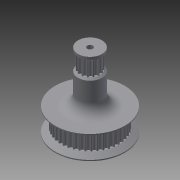
# Autodesk Inventor part: gates 42 pulley and gates 15 pulley
Saved by Autodesk Inventor 2015 (Build 190159000, 159)
## iProperties
Created: 2015-02-13
Part Number: gates 42 pulley and gates 15 pulley
Material: Generic
Document SubType Name: Modeling
Designer: robotics
Density: 1 g/cm^3
Appearance: Default
Author: robotics
Autodesk Inventor part; units mm, degrees
ref_plane "YZ Plane" through (0, 0, 0) normal (1, 0, 0) x (0, 1, 0)
ref_plane "XZ Plane" through (0, 0, 0) normal (0, 1, 0) x (-1, 0, 0)
ref_plane "XY Plane" through (0, 0, 0) normal (0, 0, 1) x (1, 0, 0)
sketch "Sketch1" plane through (0, 0, 0) normal (0, 1, 0) x (-1, 0, 0)
  circle A0 centre (0, 0) radius 32.766
  dimension "d0" = 65.532
  constraints: 1 centre point, 1 coincident
  measures "d0" diameter of A0
extrude "Extrusion1" add sketch "Sketch1" along normal blind 16.51
sketch "Sketch2" plane through (0, 16.51, 0) normal (0, 1, 0) x (1, 0, 0)
  circle A0 centre (0, 0) radius 32.766 construction
  circle A1 centre (0, 0) radius 30.6832 construction
  line L0 (0, 0) -> (-47.2853, 0) construction
  line L1 (0, 0) -> (-30.5974, -2.293) construction
  line L2 (0, 0) -> (-30.5974, 2.293) construction
  line L3 (-32.766, -0.6731) -> (-32.766, 0.6731)
  line L4 (-32.766, -0.6731) -> (-30.6758, -0.6731) construction
  line L5 (-32.766, 0.6731) -> (-32.3432, 0.6731)
  circle A2 centre (-32.3432, -2.4238) radius 1.7507 construction
  circle A3 centre (-32.3432, 2.4238) radius 1.7507 construction
  line L6 (-32.5004, 4.2179) -> (-32.2997, 5.5491)
  line L7 (-32.5004, 4.2179) -> (-32.0823, 4.1549)
  arc A4 (-32.3432, 0.6731) -> (-32.0823, 4.1549) centre (-32.3432, 2.4238) ccw
  arc A5 (-32.5004, 4.2179) -> (-32.766, 0.6731) centre (0, 0) ccw
  point P0 (-32.4, 4.8835)
  dimension "d3" = 65.532
  dimension "d4" = 61.3664
  dimension "d5" = 8.571
  dimension "d6" = 1.3462
  constraints: 16 end point, 9 point on circle, 5 centre point, 4 coincident, 4 tangent, 3 horizontal, 2 line through centre, 2 vertical, 1 equal length, 1 equal radius, 1 midpoint, 1 perpendicular, 1 symmetric about line, 5 other
  measures "d4" diameter of A1
  measures "d5" angle of L2 L1
  measures "d6" distance of L3.start L3.end
extrude "Extrusion2" cut sketch "Sketch2" against normal through all
fillet "Fillet1" radius 0.127 2 edges at (-32.7591, 8.255, -0.6731) (-32.4935, 8.255, -4.2169)
pattern_circular "Circular Pattern1" count 42 over 360 about axis through (0, 0, 0) along (0, 1, 0) of "Extrusion2", "Fillet1"
sketch "Sketch3" plane through (0, 0, 0) normal (0, 0, 1) x (1, 0, 0)
  line L0 (0, 0) -> (32.766, 0)
  line L1 (32.766, 0) -> (39.116, -3.81)
  line L2 (39.116, -3.81) -> (39.116, -4.953)
  line L3 (39.116, -4.953) -> (0, -4.953)
  line L4 (0, -4.953) -> (0, 0)
  line L5 (-1.7458, 16.51) -> (1.7458, 16.51) projected
  line L6 (0, 16.51) -> (32.766, 16.51)
  line L7 (32.766, 16.51) -> (39.116, 20.32)
  line L8 (39.116, 20.32) -> (39.116, 21.463)
  line L9 (0, 57.15) -> (0, 16.51)
  line L10 (0, 57.15) -> (11.3665, 57.15)
  line L11 (11.3665, 57.15) -> (13.4747, 55.372)
  line L12 (13.4747, 55.372) -> (13.4747, 51.0934)
  line L13 (13.4747, 51.0934) -> (13.4747, 21.463)
  line L14 (13.4747, 21.463) -> (39.116, 21.463)
  dimension "d13" = 32.766
  dimension "d14" = 3.81
  dimension "d15" = 6.35
  dimension "d16" = 4.953
  dimension "d17" = 32.766
  dimension "d18" = 3.81
  dimension "d19" = 6.35
  dimension "d22" = 4.953
  dimension "d23" = 62.103
  dimension "d24" = 11.3665
  dimension "d26" = 1.778
  dimension "d27" = 2.1082
  dimension "d54" = 13.4747
  dimension "d55" = 39.116
  constraints: 28 end point, 5 perpendicular, 2 horizontal, 1 collinear, 1 midpoint, 1 point on line, 1 vertical
  measures "d13" distance of L0.start L0.end
  measures "d14" vertical distance of L1.end L0.end
  measures "d15" horizontal distance of L1.end L0.end
  measures "d16" distance of L3.end L0.start
  measures "d17" distance of L6.start L6.end
  measures "d18" vertical distance of L7.end L6.end
  measures "d19" horizontal distance of L6.end L7.end
  measures "d22" vertical distance of L8.end L6.end
  measures "d23" distance of L9.start L3.end
  measures "d24" distance of L9.start L10.end
  measures "d26" vertical distance of L10.end L11.end
  measures "d27" horizontal distance of L10.end L11.end
  measures "d54" distance between parallel lines of L13 L9
  measures "d55" distance of L2.end L3.end
revolve "Revolution1" add sketch "Sketch3" angle 360 about axis through (0, 57.15, 0) along (0, -1, 0)
fillet "Fillet2" radius 12.7 1 edges at (-13.4747, 21.463, 0)
sketch "Sketch5" plane through (0, 57.15, 0) normal (0, 1, 0) x (1, 0, 0)
  circle A0 centre (0, 0) radius 11.3665
  dimension "d33" = 22.733
  constraints: 1 centre point, 1 coincident
  measures "d33" diameter of A0
extrude "Extrusion3" add sketch "Sketch5" along normal blind 16.51
sketch "Sketch6" plane through (0, 73.66, 0) normal (0, 1, 0) x (1, 0, 0)
  circle A0 centre (0, 0) radius 11.3665 construction
  circle A1 centre (0, 0) radius 9.2837 construction
  line L0 (0, 0) -> (0, 14.8033) construction
  line L1 (0, 0) -> (-1.9302, 9.0808) construction
  line L2 (0, 0) -> (1.9302, 9.0808) construction
  line L3 (-0.6731, 11.3665) -> (0.6731, 11.3665)
  circle A2 centre (-2.2602, 10.6332) radius 1.5871 construction
  circle A3 centre (2.2602, 10.6332) radius 1.5871 construction
  line L4 (-0.6731, 11.3665) -> (-0.6731, 9.2593) construction
  line L5 (0.6731, 11.3665) -> (0.6731, 10.6332)
  line L6 (4.0083, 10.6576) -> (5.2381, 10.11)
  line L7 (4.0083, 10.6576) -> (3.71, 9.9877)
  circle A4 centre (0, 0) radius 11.3665 construction
  arc A5 (0.6731, 10.6332) -> (3.71, 9.9877) centre (2.2602, 10.6332) ccw
  arc A6 (4.0083, 10.6576) -> (0.6731, 11.3665) centre (0.9264, 4.3583) ccw
  point P0 (4.6232, 10.3838)
  dimension "d36" = 22.733
  dimension "d37" = 18.5674
  dimension "d38" = 24
  dimension "d39" = 1.3462
  constraints: 16 end point, 9 point on circle, 6 centre point, 5 tangent, 3 coincident, 3 vertical, 2 line through centre, 1 equal length, 1 equal radius, 1 horizontal, 1 midpoint, 1 perpendicular, 1 symmetric about line, 4 other
  measures "d36" diameter of A0
  measures "d37" diameter of A1
  measures "d38" angle of L2 L1
  measures "d39" distance of L3.start L3.end
extrude "Extrusion4" cut sketch "Sketch6" against normal blind 16.51
fillet "Fillet3" radius 0.127 2 edges at (4.0002, 65.405, -10.6394) (0.6731, 65.405, -11.3466)
pattern_circular "Circular Pattern2" count 15 over 360 about axis through (0, 57.15, 0) along (0, 1, 0) of "Extrusion4", "Fillet3"
sketch "Sketch7" plane through (0, 0, 0) normal (0, 0, 1) x (1, 0, 0)
  line L0 (-1.5524, 73.66) -> (1.5524, 73.66) projected
  line L1 (0, 73.66) -> (11.3665, 73.66)
  line L2 (7.8273, 73.66) -> (9.9048, 73.66) projected
  line L3 (11.3665, 73.66) -> (13.4747, 75.438)
  line L4 (13.4747, 75.438) -> (13.4747, 78.613)
  line L5 (13.4747, 78.613) -> (0, 78.613)
  line L6 (0, 78.613) -> (0, 73.66)
  point P0 (0, 0)
  point P1 (8.3524, 73.66)
  dimension "d46" = 11.3665
  dimension "d47" = 1.778
  dimension "d48" = 2.1082
  dimension "d49" = 3.175
  constraints: 10 end point, 3 perpendicular, 1 collinear, 1 midpoint
  measures "d46" distance of L1.start L1.end
  measures "d47" vertical distance of L3.end L1.end
  measures "d48" horizontal distance of L1.end L3.end
  measures "d49" distance of L3.end L4.end
revolve "Revolution2" add sketch "Sketch7" angle 360 about axis through (0, 78.613, 0) along (0, -1, 0)
sketch "Sketch8" plane through (0, 78.613, 0) normal (0, 1, 0) x (1, 0, 0)
  circle A0 centre (0, 0) radius 3.175
  dimension "d51" = 6.35
  constraints: 1 centre point, 1 coincident
  measures "d51" diameter of A0
extrude "Extrusion5" cut sketch "Sketch8" against normal through all
equation "\"d13\" = 0.5 * d0"
equation "\"d17\" = 0.5 * d0"
equation "\"d18\" = d14"
equation "\"d19\" = d15"
equation "\"d22\" = d16"
equation "\"d47\" = d26"
equation "\"d48\" = d27"
body "Solid1"
